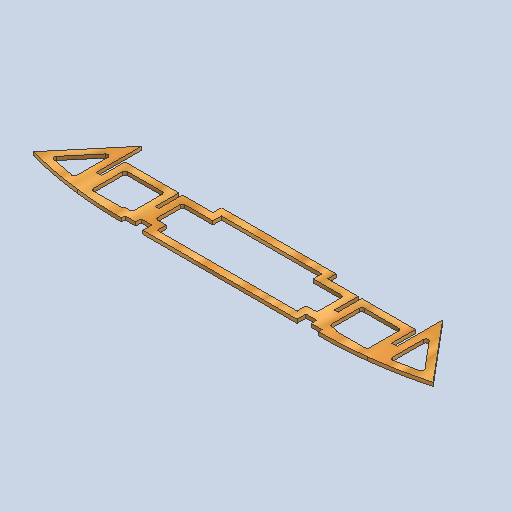
# Autodesk Inventor part: bulkhead_b1
Saved by Autodesk Inventor 2022 (Build 260153070, 153G)
## iProperties
Created: 2021-04-24
Part Number: bulkhead_b1
Material: Plywood, Sheathing, Glazed
Document SubType Name: Modeling
Designer: kardo
Density: 0.75 g/cm^3
Appearance: Plywood - New(2)
Mass: 3.95958 g
Surface Area: 75.5532 cm^2
Volume: 5.27943 cm^3
Author: kardo
Autodesk Inventor part; units mm, degrees
ref_plane "YZ Plane" through (0, 0, 0) normal (1, 0, 0) x (0, 1, 0)
ref_plane "XZ Plane" through (0, 0, 0) normal (0, 1, 0) x (-1, 0, 0)
ref_plane "XY Plane" through (0, 0, 0) normal (0, 0, 1) x (1, 0, 0)
derived "frame_outline.ipt"
sketch "bh_b1" plane through (0, -121, 0) normal (0, 1, 0) x (-1, 0, 0)
  line L0 (-34, 18.8429) -> (0, 18.8429) construction
  line L1 (-34, 18.8429) -> (-34, 23.5936) construction
  line L2 (-34, 23.5936) -> (-81, 23.5936) construction
  line L3 (-81, 23.5936) -> (-81, 7.4347) construction
  line L4 (-81, 7.4347) -> (-112.8424, 45.3829) construction
  line L5 (-81, 8.6792) -> (-111.4358, 44.9512)
  line L6 (0, 19.6429) -> (-32, 19.6429)
  line L7 (-32, 19.6429) -> (-32, 24.3936)
  line L8 (-32, 24.3936) -> (-81, 24.3936)
  line L9 (-81, 24.3936) -> (-81, 8.6792)
  line L10 (0, 52.4598) -> (0, 19.6429)
  spline S0 degree 3 poles (-81, 51.7023) (-88.6158, 50.7886) (-95.2675, 49.6052) (-104.7998, 47.5485) (-108.847, 46.5342) (-112.8424, 45.3829) knots 2.844968 2.844968 2.844968 2.844968 5.638195 5.638195 7.757395 7.757395 7.757395 7.757395
  spline S1 degree 3 poles (-55, 53.2598) (-64.4832, 53.2598) (-73.2431, 52.6329) (-81, 51.7023) knots 0 0 0 0 2.844968 2.844968 2.844968 2.844968
  spline S2 degree 3 poles (0, 53.2598) (-9.1667, 53.2598) (-18.3333, 53.2598) (-36.6667, 53.2598) (-45.8333, 53.2598) (-55, 53.2598) knots 0 0 0 0 2.75 2.75 5.5 5.5 5.5 5.5
  spline S3 degree 3 poles (-111.4358, 44.9512) (-110.6984, 45.1582) (-109.22, 45.5628) (-107.3625, 46.0458) (-105.6839, 46.4653) (-104.5611, 46.7366) (-103.435, 47.0013) (-102.6827, 47.1744) (-101.7404, 47.3867) (-100.9848, 47.5533) (-100.0386, 47.7574) (-99.263, 47.921) (-98.2716, 48.1254) (-97.4607, 48.2886) (-96.4254, 48.4919) (-95.5799, 48.6537) (-94.2862, 48.8949) (-92.9587, 49.1335) (-90.906, 49.4853) (-89.0166, 49.7903) (-86.577, 50.1591) (-84.0609, 50.5141) (-81.9694, 50.7802) (-80.9047, 50.908) knots 2.844968 2.844968 2.844968 2.844968 3.236821 3.628674 3.8246 4.11849 4.216453 4.41238 4.510343 4.706269 4.804232 5.000159 5.098122 5.294048 5.392012 5.587938 5.685901 5.979791 6.175717 6.56757 6.763496 7.155349 7.547202 7.547202 7.547202 7.547202
  spline S4 degree 3 poles (-80.9047, 50.908) (-79.6164, 51.0625) (-77.3134, 51.3194) (-74.5891, 51.5796) (-72.5078, 51.7582) (-71.1014, 51.8686) (-69.3205, 51.9947) (-67.8775, 52.0859) (-66.0518, 52.1868) (-64.5737, 52.2568) (-62.7048, 52.3303) (-61.193, 52.3777) (-59.2829, 52.4222) (-57.3527, 52.4519) (-55.7876, 52.4598) (-55, 52.4598) knots 0 0 0 0 0.474161 0.829782 0.948323 1.185403 1.303944 1.541024 1.659565 1.896646 2.015186 2.252267 2.370807 2.607888 2.844968 2.844968 2.844968 2.844968
  spline S5 degree 3 poles (-55, 52.4598) (-51.9444, 52.4598) (-46.5972, 52.4598) (-40.4861, 52.4598) (-35.9028, 52.4598) (-32.8472, 52.4598) (-29.0278, 52.4598) (-25.9722, 52.4598) (-22.1528, 52.4598) (-19.0972, 52.4598) (-15.2778, 52.4598) (-12.2222, 52.4598) (-8.4028, 52.4598) (-4.5833, 52.4598) (-1.5278, 52.4598) (0, 52.4598) knots 0 0 0 0 0.916667 1.604167 1.833333 2.291667 2.520833 2.979167 3.208333 3.666667 3.895833 4.354167 4.583333 5.041667 5.5 5.5 5.5 5.5
  point P0 (0, 0)
  point P1 (-81, 37.5562)
extrude "Extrusion1" add sketch "bh_b1" along normal blind 2
sketch "Sketch4" plane through (0, -121, 52.4598) normal (0, -1, 0) x (1, 0, 0)
  line L0 (0, 0) -> (55, 0) projected
  line L1 (0, 0) -> (55, 0) projected
  line L2 (55, 0) -> (55, -2)
  line L3 (55, -2) -> (49, -2)
  line L4 (49, -2) -> (49, -5)
  line L5 (49, -5) -> (43, -5)
  line L6 (43, -5) -> (43, 0)
  point P0 (0, -52.4598)
  dimension "d9" = 6
  dimension "d10" = 6
  dimension "d11" = 2
  dimension "d12" = 5
  constraints: 10 end point, 3 vertical, 2 horizontal, 1 point on line
  measures "d9" distance of L2.end L3.end
  measures "d10" distance of L4.end L5.end
  measures "d11" distance of L0.end L2.end
  measures "d12" distance of L5.end L6.end
sketch "Sketch2" plane through (0, -121, 52.4598) normal (0, -1, 0) x (1, 0, 0)
  line L0 (81, -43.7805) -> (81, -28.0661) projected
  line L1 (111.4358, -7.5086) -> (81, -43.7805) projected
  line L2 (81, -28.0661) -> (81, -14.9036)
  line L3 (81, -14.9036) -> (84, -14.9036)
  line L4 (84, -14.9036) -> (84, -40.2053)
  line L5 (111.4358, -7.5086) -> (81, -43.7805) projected
  point P0 (0, -52.4598)
  dimension "d3" = 3
  constraints: 6 end point, 2 point on line, 1 collinear, 1 horizontal, 1 parallel
  measures "d3" distance between parallel lines of L4 L0
extrude "Extrusion2" cut sketch "Sketch2" against normal through all
extrude "Extrusion3" cut sketch "Sketch4" against normal through all
sketch "Sketch3" plane through (0, -121, 52.4598) normal (0, -1, 0) x (1, 0, 0)
  line L0 (84, -14.9036) -> (84, -40.2053) projected
  line L1 (111.4358, -7.5086) -> (84, -40.2053) projected
  line L2 (88, -29.2153) -> (104.3123, -9.7751)
  line L3 (104.3123, -9.7751) -> (88, -6.5598)
  line L4 (88, -6.5598) -> (88, -29.2153)
  line L5 (88, -6.5598) -> (88.7736, -2.6353) construction
  line L6 (105.0858, -5.8507) -> (104.3123, -9.7751) construction
  point P0 (0, -52.4598)
  dimension "d6" = 4
  dimension "d7" = 4
  dimension "d8" = 4
  constraints: 10 end point, 3 parallel, 2 perpendicular, 3 other
  measures "d6" distance of L6.start L2.end
  measures "d7" distance between parallel lines of L1 L2
  measures "d8" distance between parallel lines of L0 L4
sketch "Sketch5" plane through (0, -121, 19.6429) normal (0, -1, 0) x (1, 0, 0)
  line L0 (55, 26.8169) -> (55, 8.7507)
  line L1 (55, 8.7507) -> (77, 8.7507)
  line L2 (77, 8.7507) -> (77, 27.6994)
  line L3 (77, 27.6994) -> (59, 27.6994)
  line L4 (55, 32.8169) -> (55, 30.8169) projected
  line L5 (81, 4.7507) -> (32, 4.7507) projected
  line L6 (81, 4.7507) -> (81, 17.9133) projected
  line L7 (77, 27.6994) -> (77, 31.6994) construction
  line L8 (49, 30.8169) -> (49, 27.8169) projected
  line L9 (59, 26.8169) -> (55, 26.8169)
  line L10 (59, 27.6994) -> (59, 26.8169)
  line L11 (55, 30.8169) -> (49, 30.8169) projected
  point P0 (0, -19.6429)
  dimension "d15" = 4
  dimension "d16" = 4
  dimension "d18" = 4
  dimension "d34" = 6
  dimension "d35" = 4
  dimension "d36" = 4
  constraints: 14 end point, 5 parallel, 2 collinear, 2 other
  measures "d15" distance between parallel lines of L6 L2
  measures "d16" distance between parallel lines of L5 L1
  measures "d18" distance of L2.end L7.end
  measures "d34" distance between parallel lines of L0 L8
  measures "d35" distance between parallel lines of L11 L9
  measures "d36" distance between parallel lines of L4 L10
sketch "Sketch6" plane through (0, -121, 19.6429) normal (0, -1, 0) x (1, 0, 0)
  line L0 (0, 0) -> (0, 32.8169) projected
  line L1 (0, 32.8169) -> (43, 32.8169) projected
  line L2 (43, 27.8169) -> (43, 32.8169) projected
  line L3 (32, 0) -> (0, 0) projected
  line L4 (32, 4.7507) -> (32, 0) projected
  line L5 (81, 4.7507) -> (32, 4.7507) projected
  line L6 (0, 28.8169) -> (39, 28.8169)
  line L7 (39, 28.8169) -> (39, 23.8169)
  line L8 (39, 23.8169) -> (45, 23.8169)
  line L9 (45, 23.8169) -> (45, 8.7507)
  line L10 (45, 8.7507) -> (28, 8.7507)
  line L11 (28, 8.7507) -> (28, 4)
  line L12 (28, 4) -> (0, 4)
  line L13 (55, 32.8169) -> (55, 30.8169) projected
  line L14 (49, 27.8169) -> (43, 27.8169) projected
  line L15 (49, 27.8169) -> (49, 30.8169) projected
  point P0 (0, -19.6429)
  dimension "d19" = 4
  dimension "d20" = 4
  dimension "d21" = 4
  dimension "d23" = 4
  dimension "d24" = 4
  dimension "d25" = 4
  dimension "d33" = 4
  constraints: 14 end point, 7 parallel, 2 point on line
  measures "d19" distance between parallel lines of L1 L6
  measures "d20" distance between parallel lines of L2 L7
  measures "d21" distance between parallel lines of L14 L8
  measures "d23" distance between parallel lines of L5 L10
  measures "d24" distance between parallel lines of L4 L11
  measures "d25" distance between parallel lines of L3 L12
  measures "d33" distance between parallel lines of L9 L15
extrude "Extrusion4" cut sketch "Sketch6" against normal through all
extrude "Extrusion5" cut sketch "Sketch5" against normal through all
extrude "Extrusion6" cut sketch "Sketch3" against normal through all
fillet "Fillet1" radius 1.3333 11 edges at (77, -120, 28.3936) (77, -120, 47.3423) (55, -120, 46.4598) (88, -120, 45.9) (55, -120, 28.3936) (88, -120, 23.2444) (104.3123, -120, 42.6846) (45, -120, 43.4598) (45, -120, 28.3936) (59, -120, 46.4598) (59, -120, 47.3423)
sketch "Sketch7" plane through (0, -121, 19.6429) normal (0, -1, 0) x (1, 0, 0)
  line L0 (81, 4.7507) -> (32, 4.7507) projected
  line L1 (49, 4.7507) -> (49, 17.9133)
  line L2 (49, 17.9133) -> (51, 17.9133)
  line L3 (51, 17.9133) -> (51, 4.7507)
  line L4 (81, 17.9133) -> (84, 17.9133) projected
  line L5 (49, 30.8169) -> (49, 27.8169) projected
  point P0 (0, -19.6429)
  dimension "d37" = 2
  constraints: 6 end point, 2 collinear, 2 point on line, 2 vertical, 1 horizontal
  measures "d37" distance between parallel lines of L1 L3
extrude "Extrusion7" cut sketch "Sketch7" against normal through all
mirror "Mirror1" about plane through (0, 0, 0) normal (1, 0, 0)
equation "\"d1\" = bulkhead_thickness"
equation "\"d9\" = cowl_liner_width"
equation "\"d10\" = cowl_insulation_width"
equation "\"d11\" = cowl_liner_thickness"
equation "\"d12\" = cowl_liner_thickness + cowl_insulation_thickness"
equation "\"d3\" = stringer_thickness"
equation "\"d6\" = inset"
equation "\"d7\" = inset"
equation "\"d8\" = inset"
equation "\"d15\" = inset"
equation "\"d16\" = inset"
equation "\"d18\" = inset"
equation "\"d34\" = inset + bulkhead_thickness"
equation "\"d35\" = inset"
equation "\"d36\" = inset"
equation "\"d19\" = inset"
equation "\"d20\" = inset"
equation "\"d21\" = inset"
equation "\"d23\" = inset"
equation "\"d24\" = inset"
equation "\"d25\" = inset"
equation "\"d33\" = inset"
equation "\"d32\" = 0.333333 * inset"
equation "\"d37\" = bulkhead_thickness"
equation "\"bulkhead_thickness\" = 2"
equation "\"cowl_liner_width\" = 6"
equation "\"cowl_insulation_width\" = 6"
equation "\"cowl_liner_thickness\" = 2"
equation "\"cowl_insulation_thickness\" = 3"
equation "\"stringer_thickness\" = 3"
equation "\"inset\" = 4"
body "Solid1"
